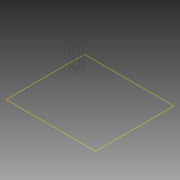
# Autodesk Inventor part: STANDOFF3
Saved by Autodesk Inventor 2015 (Build 190159000, 159)
## iProperties
Created: 2015-09-18
Part Number: STANDOFF3
Material: Generic
Description: insert part description/title
Document SubType Name: Modeling
Designer: francis
Density: 1 g/cm^3
Appearance: Default
Part Category: insert part category here and press enter to fill value
Author: francis
Autodesk Inventor part; units mm, degrees
ref_plane "YZ Plane" through (0, 0, 0) normal (1, 0, 0) x (0, 1, 0)
ref_plane "XZ Plane" through (0, 0, 0) normal (0, 1, 0) x (-1, 0, 0)
ref_plane "XY Plane" through (0, 0, 0) normal (0, 0, 1) x (1, 0, 0)
ref_plane "Work Plane1" through (0, 0, 0) normal (0, 0, 1) x (1, 0, 0)
sketch "Sketch1" plane through (0, 0, 0) normal (0, 0, 1) x (1, 0, 0)
  circle A0 centre (-35.038, 18.1476) radius 2
  circle A1 centre (-35.038, 18.1476) radius 5
  point P0 (0, 0)
  dimension "d0" = 10
  dimension "d3" = 4
  constraints: 2 centre point, 1 coincident
  measures "d0" diameter of A1
  measures "d3" diameter of A0
ref_plane "Work Plane2" through (-41.538, 5.1476, 22) normal (0, 0, -1) x (0, 1, 0)
extrude "Extrusion1" add sketch "Sketch1" along normal up to surface (22 mm away)
body "Solid1"
